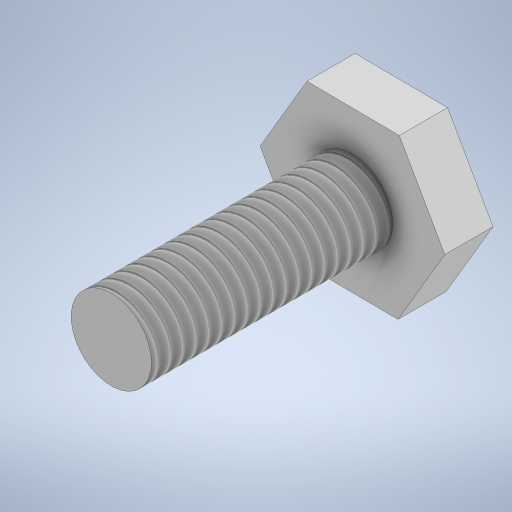
# Autodesk Inventor part: Screw
Saved by Autodesk Inventor 2024 (Build 280153000, 153)
## iProperties
Created: 2024-02-05
Part Number: Screw
Material: Generic
Document SubType Name: Modeling
Designer: Ramji Yadav
Density: 1 g/cm^3
Appearance: Default
Author: Ramji Yadav
Autodesk Inventor part; units mm, degrees
ref_plane "YZ Plane" through (0, 0, 0) normal (1, 0, 0) x (0, 1, 0)
ref_plane "XZ Plane" through (0, 0, 0) normal (0, 1, 0) x (-1, 0, 0)
ref_plane "XY Plane" through (0, 0, 0) normal (0, 0, 1) x (1, 0, 0)
sketch "Sketch1" plane through (0, 0, 0) normal (0, 0, 1) x (1, 0, 0)
  circle A0 centre (0, 0) radius 2.5
  circle A1 centre (0, 0) radius 5
  line L0 (2.8292, -5) -> (-2.9155, -4.9502)
  line L1 (-2.9155, -4.9502) -> (-5.7447, 0.0498)
  line L2 (-5.7447, 0.0498) -> (-2.8292, 5)
  line L3 (-2.8292, 5) -> (2.9155, 4.9502)
  line L4 (2.9155, 4.9502) -> (5.7447, -0.0498)
  line L5 (5.7447, -0.0498) -> (2.8292, -5)
  dimension "d0" = 5
  dimension "d1" = 10
  constraints: 12 end point, 3 coincident, 2 centre point, 13 other
  measures "d0" diameter of A0
  measures "d1" diameter of A1
extrude "Extrusion1" add sketch "Sketch1" along normal blind 3 contours A0 | A1 L5 L0 L1 L2 L3 L4 | A1 L4 L5 | A1 L3 L4 | L5 L0 A1 | A1 L2 L3 | L0 L1 A1 | A1 L1 L2
sketch "Sketch2" plane through (0, 0, 3) normal (0, 0, 1) x (1, 0, 0)
  circle A0 centre (0, 0) radius 2.5
  dimension "d4" = 5
  constraints: 1 centre point, 1 coincident
  measures "d4" diameter of A0
extrude "Extrusion2" add sketch "Sketch2" along normal blind 15
thread "Thread1" size "M5x0.8" class "6g" standard "ANSI Metric M Profile" full length
sketch "Sketch3" plane through (0, 0, 0) normal (0, 0, -1) x (-1, 0, 0)
  point P0 (0, 0)
body "Solid1"
